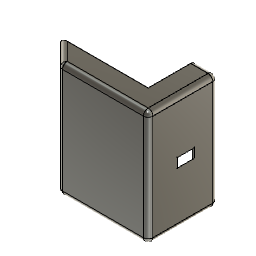
SingleSensor v7 (Autodesk Fusion 360 design; units mm, degrees)
Autodesk Fusion 360 part; units mm, degrees
sketch "Sketch1" plane through (0, 0, 0) normal (0, 1, 0) x (1, 0, 0)
  line L0 (0, 0) -> (25.8, 0)
  line L1 (25.8, 0) -> (25.8, -34.4)
  line L2 (25.8, -34.4) -> (0, -34.4)
  line L3 (0, -34.4) -> (0, 0)
  line L4 (-1, 1) -> (26.8, 1)
  line L5 (26.8, 1) -> (26.8, -35.4)
  line L6 (26.8, -35.4) -> (-1, -35.4)
  line L7 (-1, -35.4) -> (-1, 1)
  line L8 (5, 0) -> (5, 1)
  line L9 (19.8, 0) -> (19.8, 1)
  line L10 (21.8, -35.4) -> (21.8, -34.4)
  dimension "d1" = 25.8
  dimension "d2" = 34.4
  dimension "d3" = 1
  dimension "d4" = 1
  dimension "d5" = 1
  dimension "d6" = 1
  dimension "d7" = 6
  dimension "d8" = 6
  dimension "d13" = 5
  constraint horizontal L0
  constraint vertical L1
  constraint horizontal L2
  constraint vertical L3
  constraint coincident L0.start L3.end
  constraint horizontal L4
  constraint vertical L5
  constraint horizontal L6
  constraint vertical L7
  constraint coincident L0 L8.start
  constraint coincident L4 L8.end
  constraint perpendicular L4 L8
  constraint coincident L0 L9.start
  constraint coincident L4 L9.end
  constraint perpendicular L4 L9
  constraint coincident L6 L10.start
  constraint coincident L2 L10.end
  constraint perpendicular L2 L10
  measures "d1" distance of L0.start L0.end
  measures "d2" distance of L0.start L2.end
  measures "d3" distance of L2 L6
  measures "d4" distance of L3 L7
  measures "d5" distance of L0 L4
  measures "d6" distance of L1 L5
  measures "d7" distance of L1 L9
  measures "d8" distance of L7 L8
  measures "d13" distance of L5 L10
extrude "Extrude1" add sketch "Sketch1" against normal blind 6 contours L0 L2 L3 L4 L6 L7 L8 L10 | L0 L1 L2 L4 L5 L6 L9 L10 picked at (-0.666667, -22.933333) picked at (26.466667, -22.933333) makes body 1
sketch "Sketch2" plane through (0, -6, 0) normal (0, -1, 0) x (1, 0, 0)
  line L0 (25.8, 34.4) -> (25.8, 0)
  line L1 (25.8, 0) -> (19.8, 0)
  line L2 (19.8, 0) -> (19.8, -1)
  line L3 (19.8, -1) -> (26.8, -1)
  line L4 (26.8, -1) -> (26.8, 35.4)
  line L5 (26.8, 35.4) -> (-1, 35.4)
  line L6 (-1, 35.4) -> (-1, -1)
  line L7 (-1, -1) -> (5, -1)
  line L8 (5, -1) -> (5, 0)
  line L9 (5, 0) -> (0, 0)
  line L10 (0, 0) -> (0, 34.4)
  line L11 (0, 34.4) -> (25.8, 34.4)
  line L12 (-1, 35.4) -> (26.8, 35.4)
  line L13 (26.8, 35.4) -> (26.8, -1)
  line L14 (26.8, -1) -> (-1, -1)
  line L15 (-1, -1) -> (-1, 35.4)
  constraint horizontal L12
  constraint vertical L13
  constraint horizontal L14
  constraint vertical L15
  constraint coincident L3.end L4.start
  constraint coincident L5.end L6.start
extrude "Extrude2" add sketch "Sketch2" along normal blind 1 contours L0 L1 L2 L3 L4 L5 L6 L7 L8 L9 L10 L11 L12 L13 L14 L15 | L0 L1 L2 L8 L9 L10 L11 L14 picked at (26.466667, 11.466667) picked at (15.2, 22.933333) bodies 1
extrude "Extrude3" add sketch "Sketch1" along normal blind 15 contours L0 L1 L2 L4 L5 L6 L9 L10 picked at (26.466667, -22.933333) bodies 1
sketch "Sketch4" plane through (26.8, 0, 0) normal (1, 0, 0) x (0, 1, 0)
  line L0 (15, 35.4) -> (-7, 35.4)
  line L1 (-7, 35.4) -> (-7, -1)
  line L2 (-7, -1) -> (15, -1)
  line L3 (15, -1) -> (15, 35.4)
  line L4 (2.3, 18.65) -> (7.7, 18.65)
  line L5 (7.7, 18.65) -> (7.7, 15.75)
  line L6 (7.7, 15.75) -> (2.3, 15.75)
  line L7 (2.3, 15.75) -> (2.3, 18.65)
  line L8 (0, -1) -> (0, 35.4)
  dimension "d16" = 5.4
  dimension "d17" = 2.9
  dimension "d18" = 16.75
  dimension "d19" = 16.75
  dimension "d20" = 36.4
  dimension "d21" = 7.3
  dimension "d43" = 9.3
  constraint horizontal L4
  constraint vertical L5
  constraint horizontal L6
  constraint vertical L7
  measures "d16" distance of L4.start L4.end
  measures "d17" distance of L4.start L6.end
  measures "d18" distance of L0 L4
  measures "d19" distance of L2 L6
  measures "d20" distance of L0.start L2.end
  measures "d21" distance of L3 L5
  measures "d43" distance of L1 L7
extrude "Extrude4" cut sketch "Sketch4" against normal blind 1 contours L4 L5 L6 L7 picked at (5.9, 16.716667) bodies 1
sketch "Sketch5" plane through (25.8, 0, 0) normal (-1, 0, 0) x (0, -1, 0)
  line L0 (-7.7, 15.75) -> (-7.7, 18.65)
  line L1 (-7.7, 18.65) -> (-2.3, 18.65)
  line L2 (-2.3, 18.65) -> (-2.3, 15.75)
  line L3 (-2.3, 15.75) -> (-7.7, 15.75)
  line L4 (-15, 0) -> (6, 0)
  line L5 (6, 0) -> (6, 34.4)
  line L6 (6, 34.4) -> (-15, 34.4)
  line L7 (-15, 34.4) -> (-15, 0)
  line L8 (-15, 34.4) -> (-14, 34.4)
  line L9 (-14, 34.4) -> (-14, 0)
  line L10 (-14, 0) -> (-15, 0)
  line L11 (-15, 0) -> (-15, 34.4)
  line L12 (-14, 26.2) -> (-0.8, 26.2)
  line L13 (-0.8, 26.2) -> (-0.8, 8.2)
  line L14 (-0.8, 8.2) -> (-14, 8.2)
  line L15 (-14, 8.2) -> (-14, 26.2)
  line L16 (-14, 8.2) -> (-0.8, 8.2)
  line L17 (-0.8, 8.2) -> (-0.8, 7.2)
  line L18 (-0.8, 7.2) -> (-14, 7.2)
  line L19 (-14, 7.2) -> (-14, 8.2)
  line L20 (-14, 26.2) -> (-0.8, 26.2)
  line L21 (-0.8, 26.2) -> (-0.8, 27.2)
  line L22 (-0.8, 27.2) -> (-14, 27.2)
  line L23 (-14, 27.2) -> (-14, 26.2)
  line L24 (-5, 17.2) -> (-11.5, 17.2)
  line L25 (-11.5, 34.4) -> (-11.5, 0)
  line L26 (1.35, 8.3) -> (-11.35, 8.3)
  line L27 (-11.35, 8.3) -> (-11.35, 26.1)
  line L28 (-11.35, 26.1) -> (1.35, 26.1)
  line L29 (1.35, 26.1) -> (1.35, 8.3)
  line L30 (1.35, 8.3) -> (-11.35, 26.1) construction
  line L31 (-11.35, 8.3) -> (1.35, 26.1) construction
  line L32 (-11.5, 26.2) -> (-9, 26.2)
  line L33 (-9, 26.2) -> (-9, 23.7)
  line L34 (-11.5, 8.2) -> (-9, 8.2)
  line L35 (-9, 8.2) -> (-9, 10.7)
  circle A0 centre (-9, 23.7) radius 1.1
  circle A1 centre (-9, 10.7) radius 1.1
  circle A2 centre (-9, 23.7) radius 1
  circle A3 centre (-9, 10.7) radius 1
  line L36 (-11.5, 26.2) -> (-12.5, 26.2)
  line L37 (-12.5, 26.2) -> (-12.5, 8.2)
  line L38 (-12.5, 8.2) -> (-11.5, 8.2)
  line L39 (-11.5, 8.2) -> (-11.5, 26.2)
  line L40 (-0.8, 27.2) -> (-14, 27.2)
  line L41 (-14, 27.2) -> (-14, 34.4)
  line L42 (-14, 34.4) -> (-0.8, 34.4)
  line L43 (-0.8, 34.4) -> (-0.8, 27.2)
  line L44 (-0.8, 7.2) -> (-14, 7.2)
  line L45 (-14, 7.2) -> (-14, 0)
  line L46 (-14, 0) -> (-0.8, 0)
  line L47 (-0.8, 0) -> (-0.8, 7.2)
  point P0 (-5, 17.2)
  dimension "d25" = 1
  dimension "d26" = 34.4
  dimension "d29" = 13.2
  dimension "d30" = 18
  dimension "d31" = 8.2
  dimension "d32" = 8.2
  dimension "d33" = 1
  dimension "d34" = 1
  dimension "d45" = 6.5
  dimension "d56" = 12.7
  dimension "d57" = 17.8
  dimension "d58" = 2.5
  dimension "d59" = 2.5
  dimension "d60" = 2.5
  dimension "d61" = 2.5
  dimension "d62" = 2.2
  dimension "d63" = 2.2
  dimension "d64" = 2
  dimension "d65" = 2
  dimension "d89" = 1
  constraint horizontal L8
  constraint vertical L9
  constraint horizontal L10
  constraint vertical L11
  constraint coincident L6.end L7.start
  constraint horizontal L12
  constraint vertical L13
  constraint horizontal L14
  constraint vertical L15
  constraint coincident L9 L12.start
  constraint horizontal L16
  constraint vertical L17
  constraint horizontal L18
  constraint vertical L19
  constraint horizontal L20
  constraint vertical L21
  constraint horizontal L22
  constraint vertical L23
  constraint perpendicular L0 L24
  constraint coincident L6 L25.start
  constraint coincident L4 L25.end
  constraint perpendicular L4 L25
  constraint horizontal L26
  constraint perpendicular L26 L27
  constraint parallel L26 L28
  constraint parallel L27 L29
  constraint coincident L30 P0
  constraint coincident L31 P0
  constraint coincident P0 L24.start
  constraint coincident L12 L32.start
  constraint coincident L25 L32.start
  constraint perpendicular L25 L32
  constraint perpendicular L32 L33
  constraint coincident L14 L34.start
  constraint coincident L25 L34.start
  constraint perpendicular L27 L34
  constraint perpendicular L34 L35
  constraint coincident L33.end A0.centre
  constraint coincident L35.end A1.centre
  constraint concentric A1 A3
  constraint horizontal L36
  constraint vertical L37
  constraint horizontal L38
  constraint vertical L39
  constraint horizontal L40
  constraint vertical L41
  constraint horizontal L42
  constraint vertical L43
  constraint horizontal L44
  constraint vertical L45
  constraint horizontal L46
  constraint vertical L47
  measures "d25" distance of L6.end L8.end
  measures "d26" distance of L6.end L4.start
  measures "d29" distance of L12.start L12.end
  measures "d30" distance of L12.start L14.end
  measures "d31" distance of L4 L14
  measures "d32" distance of L6 L12
  measures "d33" distance of L14.end L18.end
  measures "d34" distance of L12.start L22.end
  measures "d45" distance of P0 L24.end
  measures "d56" distance of L27.end L28.end
  measures "d57" distance of L26.end L27.end
  measures "d58" distance of L32.start L32.end
  measures "d59" distance of L32.end L33.end
  measures "d60" distance of L34.start L34.end
  measures "d61" distance of L34.end L35.end
  measures "d62" diameter of A0
  measures "d63" diameter of A1
  measures "d64" diameter of A2
  measures "d65" diameter of A3
  measures "d89" distance of L32.start L36.end
extrude "Extrude5" add sketch "Sketch5" along normal blind 5 contours L4 L6 L7 L8 L9 L10 L11 L15 L19 L23 L41 L45 picked at (-14.666667, 13.866667) bodies 1
extrude "Extrude6" add sketch "Sketch5" along normal blind 5 contours L9 L14 L16 L18 L19 L25 L38 L44 | L14 L16 L17 L18 L25 L34 L44 | L9 L12 L20 L22 L23 L25 L36 L40 | L12 L20 L21 L22 L25 L32 L40 picked at (-12.666667, 7.533333) picked at (-7.1, 7.533333) picked at (-12.666667, 26.866667) picked at (-7.1, 26.866667) bodies 1
extrude "Extrude7" cut 1 faces at (20.8, 14.666667, 13.866667) along direction (1, 0, 0) blind 1 on bodies 1 bodies 1
chamfer "Chamfer3" distance 1 angle 45 4 edges at (25.8, 5, 18.65) (25.8, 2.3, 17.2) (25.8, 5, 15.75) (25.8, 7.7, 17.2) on bodies 1
chamfer "Chamfer4" distance 2 angle 63.4 3 edges at (25.8, 14, 30.8) (25.8, 14, 17.2) (25.8, 14, 3.6) measured on face at (25.8, -3.5666, 16.3834) measured on face at (25.8, -3.5666, 16.3834) measured on face at (25.8, -3.5666, 16.3834) on bodies 1
extrude "Extrude8" add 2 faces at (21.8, 14.666667, 20.533333) (21.802031, 14, 20.2) along direction (-1, 0, 0) blind 2 on bodies 1 bodies 1
chamfer "Chamfer5" distance 6 angle 45 2 edges at (19.8, 0.8, 26.7) (19.8, 0.8, 7.7) measured on face at (19.8, 14.666667, 20.2) measured on face at (19.8, 14.666667, 20.2) on bodies 1
extrude "Extrude9" add 1 faces at (23.7996, 6.532933, 27.2) along direction (0, 0, 1) blind 7.5 on bodies 1 bodies 1
extrude "Extrude10" add 1 faces at (23.7996, 6.532933, 7.2) along direction (0, 0, -1) blind 7.5 on bodies 1 bodies 1
sketch "Sketch6" plane through (25.8, 0, 0) normal (-1, 0, 0) x (0, -1, 0)
extrude "Extrude11" add sketch "Sketch5" along normal blind 3 contours A2 | A3 picked at (-8.64532, 23.508033) picked at (-8.787009, 10.534198) bodies 1
revolve "Revolve1" add 1 faces at (-1, -2.333333, 23.266667) angle 45 about axis through (-1, -7, 35.4) along (0, 0, 1) on bodies 1 bodies 1
delete_face "DeleteFace1" 1 faces at (0, -2, 22.933333) on bodies 1
sketch "Sketch7" plane through (0, 0, 0) normal (0, 0, 1) x (-1, 0, 0)
  line L0 (2, 6) -> (-5, 6)
  line L1 (-5, 6) -> (-5, 0)
  line L2 (-5, 0) -> (1, 0)
  arc A0 (1, 0) -> (5.949747, 2.050253) centre (1, 7) ccw
  line L3 (5.949747, 2.050253) -> (2, 6)
  line L4 (1, 7) -> (0, 7)
  line L5 (5.949747, 2.050253) -> (8.002564, -0.002564)
  line L6 (8.002564, -0.002564) -> (0, 0)
  line L7 (8.002564, -0.002564) -> (7.002564, -0.002243)
  line L8 (7.002564, -0.002243) -> (0, 7)
  dimension "d69" = 1
  dimension "d70" = 1
  constraint coincident A0.centre L4.start
  constraint parallel L0 L4
  constraint parallel L3 L5
  constraint coincident L6.end origin
  constraint parallel L6 L7
  measures "d69" distance of A0.centre L4.end
extrude "Extrude12" add sketch "Sketch7" along normal blind 35.4 contours L0 A0 L3 L8 | A0 L5 L6 L7 L8 picked at (2.808204, 4.525228) picked at (6.984958, 0.681815) bodies 1
extrude "Extrude13" add sketch "Sketch7" against normal blind 1 separate body contours L2 A0 L6 L8 picked at (5.690114, 0.865411) makes body 2
sketch "Sketch8" plane through (0, 0, 35.4) normal (0, 0, 1) x (-1, 0, 0)
  line L0 (8.002564, -0.002564) -> (1, 7)
  line L1 (1, 7) -> (-26.8, 7)
  line L2 (-26.8, 7) -> (-26.8, -15)
  line L3 (-26.8, -15) -> (-19.8, -15)
  line L4 (-19.8, -15) -> (-19.8, 0)
  line L5 (-19.8, 0) -> (1, 0)
  arc A0 (1, 0) -> (5.424566, 1.575683) centre (1, 7) ccw
  line L6 (5.424566, 1.575683) -> (7.002564, -0.002243)
  line L7 (7.002564, -0.002243) -> (8.002564, -0.002564)
  line L8 (8.002564, -0.002564) -> (0, 0)
  constraint coincident L8.end origin
extrude "Extrude14" add sketch "Sketch8" against normal blind 1 contours L5 A0 L6 L8 picked at (5.690114, 0.865411) bodies 1
extrude "Extrude15" add sketch "Sketch7" against normal blind 1 contours A0 L5 L6 L7 L8 picked at (6.984958, 0.681815) bodies 1 2
sketch "Sketch9" plane through (19.8, 0, 0) normal (-1, 0, 0) x (0, -1, 0)
  line L0 (-15, -1) -> (6, -1)
  line L1 (6, -1) -> (6, 0)
  line L2 (6, 0) -> (-6.8, 0)
  line L3 (-6.8, 0) -> (-6.8, 8.2)
  line L4 (-6.8, 8.2) -> (-14, 8.2)
  line L5 (-14, 8.2) -> (-14, 26.2)
  line L6 (-14, 26.2) -> (-6.8, 26.2)
  line L7 (-6.8, 26.2) -> (-6.8, 34.4)
  line L8 (-6.8, 34.4) -> (0, 34.4)
  line L9 (0, 34.4) -> (0, 35.4)
  line L10 (0, 35.4) -> (-15, 35.4)
  line L11 (-15, 35.4) -> (-15, -1)
  line L12 (-6.8, 26.2) -> (-14, 26.2)
  line L13 (-14, 26.2) -> (-14, 34.4)
  line L14 (-14, 34.4) -> (-6.8, 34.4)
  line L15 (-6.8, 34.4) -> (-6.8, 26.2)
  line L16 (-6.8, 8.2) -> (-14, 8.2)
  line L17 (-14, 8.2) -> (-14, 0)
  line L18 (-14, 0) -> (-6.8, 0)
  line L19 (-6.8, 0) -> (-6.8, 8.2)
  constraint horizontal L12
  constraint vertical L13
  constraint horizontal L14
  constraint vertical L15
  constraint coincident L6.end L7.start
  constraint horizontal L16
  constraint vertical L17
  constraint horizontal L18
  constraint vertical L19
  constraint coincident L3.end L4.start
extrude "Extrude16" cut sketch "Sketch9" against normal blind 6 contours L6 L7 L12 L13 L14 L15 picked at (-9.2, 31.666667) bodies 1
extrude "Extrude17" cut sketch "Sketch9" against normal blind 6 contours L3 L4 L16 L17 L18 L19 picked at (-9.2, 5.466667) bodies 1
extrude "Extrude18" cut 1 faces at (24.468697, 13.333333, 8.2) along direction (0, 0, 1) blind 19 on bodies 1 bodies 1
extrude "Extrude19" cut 2 faces at (21.8, 6.8, 28.933333) (21.8, 6.8, 2.733333) along direction (0, -1, 0) blind 6 on bodies 1 bodies 1
extrude "Extrude20" add sketch "Sketch5" along normal blind 3 contours L14 L16 L17 L18 L25 L34 L44 | L12 L20 L21 L22 L25 L32 L40 picked at (-7.1, 7.533333) picked at (-7.1, 26.866667) bodies 1
fillet "Fillet2" radius 1.5 11 edges at (-4.501282, -3.498718, -1) (12.9, -7, -1) (-1, -7, 17.2) (-4.501282, -3.498718, 35.4) (12.9, -7, 35.4) (26.8, -7, 17.2) (26.8, 4, 35.4) (26.8, 15, 17.2) (23.3, 15, 35.4) (23.3, 15, -1) (26.8, 4, -1) on bodies 1
extrude "Extrude22" add 1 faces at (5, -3.833333, -0.333333) along direction (1, 0, 0) blind 15 on bodies 1 bodies 1
revolve "Revolve2" add 1 faces at (-5.001724, -1.998504, 11.466667) angle 15 about axis through (-1.000046, -6, 0) along (0, 0, -1) on bodies 1 bodies 1
extrude "Extrude23" cut 1 faces at (-5.192929, 0.7687, 34.4) along direction (0, 0, -1) blind 35 on bodies 1 bodies 1
extrude "Extrude24" cut 4 faces at (22.8, 4.366667, 7.533333) (22.8, 8.639327, 10.335183) (22.8, 9.255437, 23.975295) (22.8, 4.366667, 26.533333) along direction (1, 0, 0) blind 1 on bodies 1 bodies 1
extrude "Extrude25" add 2 faces at (25.133333, 11.5, 7.866667) (25.133333, 11.5, 26.866667) along direction (0, 1, 0) blind 3 on bodies 1 bodies 1
extrude "Extrude26" add sketch "Sketch5" along normal blind 5 contours L4 L9 L18 L25 L44 L45 L46 | L4 L18 L25 L44 L46 L47 | L6 L9 L22 L25 L40 L41 L42 | L6 L22 L25 L40 L42 L43 picked at (-13.166667, 4.8) picked at (-7.933333, 4.8) picked at (-13.166667, 32) picked at (-4.366667, 29.6) bodies 1
extrude "Extrude27" add 2 faces at (20.8, 9.6, 32) (20.8, 5.2, 4.8) along direction (-1, 0, 0) blind 0.5 on bodies 1 bodies 1
